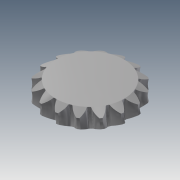
# Autodesk Inventor part: Worm Gear
Saved by Autodesk Inventor 2018 (Build 220112000, 112)
## iProperties
Created: 2019-02-07
Part Number: Worm Gear
Material: Steel, Mild
Document SubType Name: Modeling
Designer: Tsche
Categories: <?xml version="1.0" encoding="UTF-16"?> <MemberInstance><Categories><FamilyTemplate><FamilyTemplateParameter ValueType="xs:double" Id="1" ObjectReferenceKey="da_z" ObjectType="kUserParameterObject"/><FamilyTemplateParameter ValueType="xs:double" Id="2" ObjectReferenceKey="da_b" ObjectType="kUserParameterObject"/><FamilyTemplateParameter ValueType="xs:double" Id="3" ObjectReferenceKey="da_beta" ObjectType="kUserParameterObject"/><FamilyTemplateParameter ValueType="xs:double" Id="4" ObjectReferenceKey="da_m" ObjectType="kUserParameterObject"/><FamilyTemplateParameter ValueType="xs:double" Id="5" ObjectReferenceKey="da_alpha" ObjectType="kUserParameterObject"/><FamilyTemplateParameter ValueType="xs:double" Id="6" ObjectReferenceKey="da_da" ObjectType="kUserParameterObject"/><FamilyTemplateParameter ValueType="xs:double" Id="7" ObjectReferenceKey="da_aw" ObjectType="kUserParameterObject"/><FamilyTemplateParameter ValueType="xs:double" Id="8" ObjectReferenceKey="da_px" ObjectType="kUserParameterObject"/><FamilyTemplateParameter ValueType="xs:double" Id="9" ObjectReferenceKey="da_d" ObjectType="kUserParameterObject"/><FamilyTemplateParameter ValueType="xs:double" Id="10" ObjectReferenceKey="da_dae" ObjectType="kUserParameterObject"/><FamilyTemplateParameter ValueType="xs:double" Id="11" ObjectReferenceKey="da_fi" ObjectType="kUserParameterObject"/><FamilyTemplateParameter ValueType="xs:string" Id="12" ObjectReferenceKey="EAIAABAAAAAWFwAAAAAAAIAAAAAAAAAA" ObjectType="83910656" SubObjectId="SurfaceGeometry"/></FamilyTemplate><ParamToTemplateMap><ParamToTemplate CategoryParameter="//CategoryParameter[@InternalName='046C89C9-8512-4d59-83FE-43B91F4F132A']" TemplateParameter="1"/><ParamToTemplate CategoryParameter="//CategoryParameter[@InternalName='2552DF32-E462-4b46-AEBF-C6C7768E72AC']" TemplateParameter="2"/><ParamToTemplate CategoryParameter="//CategoryParameter[@InternalName='C9EE641D-15FC-4fae-A226-E94C4372FDD7']" TemplateParameter="3"/><ParamToTemplate><ParamToTemplate CategoryParameter="//CategoryParameter[@InternalName='00B6519A-459B-49c7-AD84-2E56D39A5744']" ConstantValue="0.000000"/></ParamToTemplate><ParamToTemplate><ParamToTemplate CategoryParameter="//CategoryParameter[@InternalName='04B31F0E-C7A6-4894-AA32-9629BEFACF47']" ConstantValue="1.000000"/></ParamToTemplate><ParamToTemplate><ParamToTemplate CategoryParameter="//CategoryParameter[@InternalName='43CBEC2E-7847-49e7-A936-2F7889FCB2D9']" ConstantValue="0.200000"/></ParamToTemplate><ParamToTemplate><ParamToTemplate CategoryParameter="//CategoryParameter[@InternalName='B1EFC894-105D-4ebd-86BF-FA20ED196853']" ConstantValue="0.300000"/></ParamToTemplate><ParamToTemplate><ParamToTemplate CategoryParameter="//CategoryParameter[@InternalName='51175063-3D10-4879-93E8-6246FE8B403D']" ConstantValue="2060000000.000000"/></ParamToTemplate><ParamToTemplate><ParamToTemplate CategoryParameter="//CategoryParameter[@InternalName='A3A52E27-4454-46a9-B0BD-C932399B70AF']" ConstantValue="0.300000"/></ParamToTemplate><ParamToTemplate CategoryParameter="//CategoryParameter[@InternalName='91B76062-C214-41d9-B1B9-14D2AB99603D']" TemplateParameter="4"/><ParamToTemplate CategoryParameter="//CategoryParameter[@InternalName='2D373A89-B862-43d6-8D0B-0CBF12AB9F6C']" TemplateParameter="5"/><ParamToTemplate CategoryParameter="//CategoryParameter[@InternalName='37777632-D6A2-4fac-9D53-DB8ACD95C989']" TemplateParameter="6"/><ParamToTemplate CategoryParameter="//CategoryParameter[@InternalName='FD1017F1-B727-4f7e-9707-0F86F1FF9423']" TemplateParameter="7"/><ParamToTemplate CategoryParameter="//CategoryParameter[@InternalName='3BF567DA-17EF-48d8-80EA-D119B07F6463']" TemplateParameter="8"/><ParamToTemplate CategoryParameter="//CategoryParameter[@InternalName='BF5A1E7E-5373-4a22-AAD3-F583781FCF3C']" TemplateParameter="9"/><ParamToTemplate CategoryParameter="//CategoryParameter[@InternalName='2A200944-5A8C-41ca-B96E-8520D2E510F1']" TemplateParameter="10"/><ParamToTemplate CategoryParameter="//CategoryParameter[@InternalName='E77AC4FD-7B43-4566-B0ED-7CA70B976BC8']" TemplateParameter="11"/><ParamToTemplate><ParamToTemplate CategoryParameter="//CategoryParameter[@InternalName='D4F72237-D604-435a-AD0B-F738B7463A00']" ConstantValue="110.000000"/></ParamToTemplate><ParamToTemplate><ParamToTemplate CategoryParameter="//CategoryParameter[@InternalName='9E1B4470-B2D3-4ff1-B813-535BB4CDF51A']" ConstantValue="2000000.000000"/></ParamToTemplate><ParamToTemplate><ParamToTemplate CategoryParameter="//CategoryParameter[@InternalName='A7A89E9A-52E6-4d4f-86CF-A81914F22AA4']" ConstantValue="250000000.000000"/></ParamToTemplate><ParamToTemplate><ParamToTemplate CategoryParameter="//CategoryParameter[@InternalName='B02FABAC-469F-4ad8-A219-DB4578299DF6']" ConstantValue="250000000.000000"/></ParamToTemplate><ParamToTemplate><ParamToTemplate CategoryParameter="//CategoryParameter[@InternalName='E6981962-40D5-4343-A0AD-C263FCC47E10']" ConstantValue="9.000000"/></ParamToTemplate><ParamToTemplate><ParamToTemplate CategoryParameter="//CategoryParameter[@InternalName='B958E99F-2BCD-4955-8634-793EB7B37B89']" ConstantValue="8.000000"/></ParamToTemplate><ParamToTemplate><ParamToTemplate CategoryParameter="//CategoryParameter[@InternalName='4AD49A87-569D-440f-A541-E3B52A6A9DCE']" ConstantValue="1200.000000"/></ParamToTemplate><ParamToTemplate><ParamToTemplate CategoryParameter="//CategoryParameter[@InternalName='4E5813A0-330D-4b41-BE23-D880B01A1D55']" ConstantValue="1650000.000000"/></ParamToTemplate><ParamToTemplate><ParamToTemplate CategoryParameter="//CategoryParameter[@InternalName='19EB8C86-AA88-4253-B4AA-2F5DF1CE171A']" ConstantValue="6000.000000"/></ParamToTemplate><ParamToTemplate CategoryParameter="//CategoryParameter[@InternalName='27C3BAF2-7550-4e4b-AE2C-0DB134B7D9B7']" TemplateParameter="12"/></ParamToTemplateMap><Category DisplayName="Gear" InternalName="DC85795E-93AB-48d5-8EEE-5A27447B64BD" Mnemonic="Gear"><CategoryParameter DisplayName="z" InternalName="046C89C9-8512-4d59-83FE-43B91F4F132A" Mnemonic="z"/><CategoryParameter DisplayName="b|.2|" InternalName="2552DF32-E462-4b46-AEBF-C6C7768E72AC" Mnemonic="b"/><CategoryParameter DisplayName="||b|" InternalName="C9EE641D-15FC-4fae-A226-E94C4372FDD7" Mnemonic="beta"/><CategoryParameter DisplayName="x" InternalName="00B6519A-459B-49c7-AD84-2E56D39A5744" Mnemonic="x"/><CategoryParameter DisplayName="a*" InternalName="04B31F0E-C7A6-4894-AA32-9629BEFACF47" Mnemonic="a"/><CategoryParameter DisplayName="c*" InternalName="43CBEC2E-7847-49e7-A936-2F7889FCB2D9" Mnemonic="c"/><CategoryParameter DisplayName="r|.f|*" InternalName="B1EFC894-105D-4ebd-86BF-FA20ED196853" Mnemonic="rf"/><CategoryParameter DisplayName="E" InternalName="51175063-3D10-4879-93E8-6246FE8B403D" Mnemonic="E"/><CategoryParameter DisplayName="||m|" InternalName="A3A52E27-4454-46a9-B0BD-C932399B70AF" Mnemonic="mi"/><Category DisplayName="WormGear" InternalName="1B25C7EF-093B-4025-B3D3-619CD2A4550C" Mnemonic="WormGear"><CategoryParameter DisplayName="m" InternalName="91B76062-C214-41d9-B1B9-14D2AB99603D" Mnemonic="m"/><CategoryParameter DisplayName="||a|" InternalName="2D373A89-B862-43d6-8D0B-0CBF12AB9F6C" Mnemonic="alpha"/><CategoryParameter DisplayName="d|.a|" InternalName="37777632-D6A2-4fac-9D53-DB8ACD95C989" Mnemonic="da"/><CategoryParameter DisplayName="a|.w|" InternalName="FD1017F1-B727-4f7e-9707-0F86F1FF9423" Mnemonic="aw"/><CategoryParameter DisplayName="p|.x|" InternalName="3BF567DA-17EF-48d8-80EA-D119B07F6463" Mnemonic="px"/><CategoryParameter DisplayName="d" InternalName="BF5A1E7E-5373-4a22-AAD3-F583781FCF3C" Mnemonic="d"/><CategoryParameter DisplayName="dae" InternalName="2A200944-5A8C-41ca-B96E-8520D2E510F1" Mnemonic="dae"/><CategoryParameter DisplayName="||d|" InternalName="E77AC4FD-7B43-4566-B0ED-7CA70B976BC8" Mnemonic="fi"/><CategoryParameter DisplayName="VHV" InternalName="D4F72237-D604-435a-AD0B-F738B7463A00" Mnemonic="VHV"/><CategoryParameter DisplayName="||s||.Hlim|" InternalName="9E1B4470-B2D3-4ff1-B813-535BB4CDF51A" Mnemonic="sHlim"/><CategoryParameter DisplayName="N|.Flim|" InternalName="A7A89E9A-52E6-4d4f-86CF-A81914F22AA4" Mnemonic="NFlim"/><CategoryParameter DisplayName="N|.Hlim|" InternalName="B02FABAC-469F-4ad8-A219-DB4578299DF6" Mnemonic="NHlim"/><CategoryParameter DisplayName="q|.F|" InternalName="E6981962-40D5-4343-A0AD-C263FCC47E10" Mnemonic="qF"/><CategoryParameter DisplayName="q|.H|" InternalName="B958E99F-2BCD-4955-8634-793EB7B37B89" Mnemonic="qH"/><CategoryParameter DisplayName="v|.max|" InternalName="4AD49A87-569D-440f-A541-E3B52A6A9DCE" Mnemonic="maxv"/><CategoryParameter DisplayName="S|.n|" InternalName="4E5813A0-330D-4b41-BE23-D880B01A1D55" Mnemonic="Sn"/><CategoryParameter DisplayName="K|.w|" InternalName="19EB8C86-AA88-4253-B4AA-2F5DF1CE171A" Mnemonic="Kw"/><CategoryParameter DisplayName="PitchDiameter" InternalName="27C3BAF2-7550-4e4b-AE2C-0DB134B7D9B7" Mnemonic="IDS_PITCHDIAM"/></Category></Category></Categories></MemberInstance>
Density: 7.86 g/cm^3
Appearance: Steel
CustomPartVersion: 1
Author: Tsche
Autodesk Inventor part; units mm, degrees
sketch "Sketch9" plane through (0, 0, 0) normal (0, 0, 1) x (1, 0, 0)
  spline S0 degree 4 poles (-1.8496, 10.8434) (-1.7998, 10.7978) (-1.7009, 10.7058) (-1.5459, 10.5544) (-1.3329, 10.3239) (-1.1209, 10.0648) (-0.9158, 9.786) (-0.7302, 9.464) (-0.6035, 9.2436) (-0.4689, 8.8382) (-0.423, 8.7684) (-0.3393, 8.6727) (-0.2622, 8.6399) (-0.1993, 8.6478) (-0.1698, 8.6483) knots 0 0 0 0 0 0.083363 0.166726 0.277875 0.389023 0.500167 0.611302 0.70854 0.791872 0.861267 0.916769 1 1 1 1 1
  line L0 (-0.5286, 8.6413) -> (0.1889, 8.6554) construction
  arc A0 (0.0361, 8.5685) -> (-0.3725, 8.5605) centre (-0.1641, 8.3574) ccw construction
  circle A1 centre (0, 0) radius 8.65 construction
  circle A2 centre (0, 0) radius 8.6603 construction
  circle A3 centre (0, 0) radius 10 construction
  circle A4 centre (0, 0) radius 11 construction
  line L1 (0, 0) -> (0, 11) construction
  line L2 (-0.216, 10.9979) -> (0, 0) construction
  line L3 (-1.8496, 10.8434) -> (-2.5, 11.4389)
  line L4 (-2.1516, 11.1199) -> (-1.5476, 10.5669) construction
  arc A5 (-1.6113, 10.6188) -> (-2.0943, 11.061) centre (-9.4861, 2.5022) ccw construction
  line L5 (-2.5, 11.4389) -> (-2.5, 12.998)
  line L6 (-2.5, 12.998) -> (0, 12.998)
  arc A6 (0, 8.65) -> (-0.1698, 8.6483) centre (0, 0) ccw
  line L7 (1.8496, 10.8434) -> (2.5, 11.4389)
  line L8 (2.5, 11.4389) -> (2.5, 12.998)
  line L9 (2.5, 12.998) -> (0, 12.998)
  arc A7 (0.1698, 8.6483) -> (0, 8.65) centre (0, 0) ccw
  spline S1 degree 4 poles (1.8496, 10.8434) (1.7998, 10.7978) (1.7009, 10.7058) (1.5459, 10.5544) (1.3329, 10.3239) (1.1209, 10.0648) (0.9158, 9.786) (0.7302, 9.464) (0.6035, 9.2436) (0.4689, 8.8382) (0.423, 8.7684) (0.3393, 8.6727) (0.2622, 8.6399) (0.1993, 8.6478) (0.1698, 8.6483) knots 0 0 0 0 0 0.083363 0.166726 0.277875 0.389023 0.500167 0.611302 0.70854 0.791872 0.861267 0.916769 1 1 1 1 1
  line L10 (0.5286, 8.6413) -> (-0.1889, 8.6554) construction
  line L11 (2.1516, 11.1199) -> (1.5476, 10.5669) construction
  arc A8 (0.3725, 8.5605) -> (-0.0361, 8.5685) centre (0.1641, 8.3574) ccw construction
  arc A9 (2.0943, 11.061) -> (1.6113, 10.6188) centre (9.4861, 2.5022) ccw construction
  line L12 (-2.5, 12.998) -> (-2.5, 17) construction
  line L13 (-2.5, 17) -> (2.5, 17) construction
  line L14 (2.5, 17) -> (2.5, 12.998) construction
  constraints: 1 other
ref_plane "Tooth Plane" through (0, -10, 0) normal (-0.071247, 0, 0.9974587) x (0, 1, 0)
sketch "Base Body Sketch" plane through (0, 0, 0) normal (1, 0, 0) x (0, 1, 0)
  line L0 (0, -8.4) -> (0, 8.4) projected
  line L1 (0, 2.5) -> (9.035, 2.5)
  line L2 (9.035, 2.5) -> (11.5, 1.0768)
  line L3 (-4.6, 0) -> (27.6, 0) construction
  circle A0 centre (17, 0) radius 6
  line L4 (11.5, 1.0768) -> (11.5, -1.0768)
  line L5 (0, -2.5) -> (9.035, -2.5)
  line L6 (0, 2.5) -> (0, -2.5)
  line L7 (9.035, -2.5) -> (11.5, -1.0768)
  dimension "d87" = 23
  dimension "d89" = 12
  dimension "d92" = 5
  dimension "d93" = 17
  dimension "d119" = 30
  dimension "d122" = 9.035
  constraints: 14 end point, 3 symmetric about line, 2 perpendicular, 1 centre point, 1 collinear, 1 point on line
  measures "d87" diameter of L4 L0
  measures "d89" diameter of A0
  measures "d92" distance of L1.start L5.start
  measures "d93" distance from line of A0.centre L6
  measures "d119" angle of L1 L2
  measures "d122" distance of L1.start L1.end
revolve "Base Body" add sketch "Base Body Sketch" angle 360 about axis through (0, 0, 0) along (0, 0, 1) picked at (11.3385, 0.1438) contours L0 L1 L2 A0 L7 L5 | A0 L2 L4 L7
revolve "Base Body2" cut sketch "Base Body Sketch" angle 360 about axis through (0, 0, 0) along (0, 0, 1) contours L7 L4 L2 A0 | A0 L2 L4 L7
sketch "Tooth Sketch" plane through (0, -10, 0) normal (-0.071247, 0, 0.9974587) x (0, 1, 0)
  line L0 (10, 2.2608) -> (10, -2.2608) projected
  line L1 (-8.64, 0) -> (2.84, 0) projected
  line L2 (-7, 1.6149) -> (-7, -1.6149)
  line L3 (-7, -1.6149) -> (-1.2, -1.6149)
  line L4 (-1.2, -1.6149) -> (1.2, -0.7413)
  line L5 (1.2, -0.7413) -> (1.2, 0)
  line L6 (1.2, 0.7413) -> (-1.2, 1.6149)
  line L7 (-1.2, 1.6149) -> (-7, 1.6149)
  line L8 (1.2, 0.7413) -> (1.2, 0)
  line L9 (0, 0) -> (0, -1.1781) construction
  dimension "d38" = 17
  dimension "d39" = 20
  dimension "d40" = 5.8
  dimension "d41" = 7
  dimension "d42" = 1.1781
  constraints: 16 end point, 4 perpendicular, 3 equal length, 2 point on line, 1 midpoint, 1 parallel, 1 vertical
  measures "d38" distance between parallel lines of L0 L2
  measures "d39" angle of L6 L7
  measures "d40" distance of L6.end L2.start
  measures "d41" distance between parallel lines of L2 L9
  measures "d42" distance of L9.start L9.end
sketch "Sketch8" plane through (0, 0, 2.5) normal (0, 0, 1) x (1, 0, 0)
  circle A0 centre (0, 0) radius 9.035 projected
  circle A1 centre (0, 0) radius 10
  dimension "d77" = 20
  constraints: 1 centre point, 1 coincident
  measures "d77" diameter of A1
sketch "involute_tooth" plane through (0, 0, 0) normal (0, 0, 1) x (1, 0, 0)
  spline S0 degree 4 poles (-1.6363, 10.8776) (-1.5874, 10.831) (-1.4904, 10.7371) (-1.3384, 10.5827) (-1.1299, 10.3481) (-0.9231, 10.0849) (-0.7235, 9.8021) (-0.5442, 9.4765) (-0.4219, 9.2536) (-0.2952, 8.8457) (-0.2508, 8.775) (-0.169, 8.6777) (-0.0925, 8.6433) (-0.0295, 8.65) (0, 8.65) knots 0 0 0 0 0 0.083363 0.166726 0.277875 0.389023 0.500167 0.611302 0.70854 0.791872 0.861267 0.916769 1 1 1 1 1
  line L0 (-0.3588, 8.65) -> (0.3588, 8.65) construction
  arc A0 (0.2043, 8.5662) -> (-0.2043, 8.5662) centre (0, 8.359) ccw construction
  circle A1 centre (0, 0) radius 8.65 construction
  circle A2 centre (0, 0) radius 8.6603 construction
  circle A3 centre (0, 0) radius 10 construction
  circle A4 centre (0, 0) radius 11 construction
  line L1 (0, 0) -> (0.216, 10.9979) construction
  line L2 (0, 11) -> (0, 0) construction
  line L3 (-1.6363, 10.8776) -> (-2.2749, 11.4857)
  line L4 (-1.9329, 11.16) -> (-1.3398, 10.5952) construction
  arc A5 (-1.4025, 10.6484) -> (-1.8767, 11.1) centre (-9.4352, 2.688) ccw construction
  line L5 (-2.2749, 11.4857) -> (-2.2443, 13.0446)
  line L6 (-2.2443, 13.0446) -> (0.2552, 12.9955)
  arc A6 (0.1698, 8.6483) -> (0, 8.65) centre (0, 0) ccw
  line L7 (2.0621, 10.805) -> (2.7241, 11.3876)
  line L8 (2.7241, 11.3876) -> (2.7547, 12.9464)
  line L9 (2.7547, 12.9464) -> (0.2552, 12.9955)
  arc A7 (0.3396, 8.6433) -> (0.1698, 8.6483) centre (0, 0) ccw
  spline S1 degree 4 poles (2.0621, 10.805) (2.0114, 10.7604) (1.9108, 10.6704) (1.7529, 10.522) (1.5353, 10.2958) (1.3183, 10.0408) (1.1078, 9.7662) (0.9158, 9.4479) (0.7848, 9.2299) (0.6423, 8.8273) (0.5951, 8.7584) (0.5095, 8.6644) (0.4318, 8.633) (0.3691, 8.6422) (0.3396, 8.6433) knots 0 0 0 0 0 0.083363 0.166726 0.277875 0.389023 0.500167 0.611302 0.70854 0.791872 0.861267 0.916769 1 1 1 1 1
  line L10 (0.6981, 8.6292) -> (-0.0189, 8.6574) construction
  line L11 (2.3695, 11.0755) -> (1.7547, 10.5345) construction
  arc A8 (0.5405, 8.5515) -> (0.1321, 8.5676) centre (0.3282, 8.3526) ccw construction
  arc A9 (2.3111, 11.0178) -> (1.8194, 10.5851) centre (9.5334, 2.3155) ccw construction
  line L12 (-2.2443, 13.0446) -> (-2.1657, 17.0458) construction
  line L13 (-2.1657, 17.0458) -> (2.8333, 16.9476) construction
  line L14 (2.8333, 16.9476) -> (2.7547, 12.9464) construction
  point P0 (0.3349, 9.3778)
  point P1 (-1.1477, 10.3628)
  point P2 (-0.9274, 10.0843)
  point P3 (-0.7266, 9.7915)
  point P4 (-0.549, 9.4841)
  point P5 (-0.4003, 9.1618)
  point P6 (-0.2776, 8.8289)
  point P7 (-0.2307, 8.7536)
  point P8 (-0.1685, 8.6905)
  point P9 (-0.0886, 8.6532)
  point P10 (1.5536, 10.3097)
  point P11 (1.3226, 10.0401)
  point P12 (1.1105, 9.7554)
  point P13 (0.9209, 9.4553)
  point P14 (0.7597, 9.139)
  point P15 (0.624, 8.8112)
  point P16 (0.5742, 8.7378)
  point P17 (0.5096, 8.6772)
  point P18 (0.4283, 8.6431)
  dimension "d97" = 1.125
  dimension "d98" = 2.5
  dimension "d99" = 17
  constraints: 30 end point, 24 symmetric about line, 15 point on circle, 9 centre point, 6 midpoint, 3 collinear, 2 horizontal, 2 parallel, 2 point on line, 1 coincident, 1 perpendicular, 1 tangent, 1 vertical, 54 other
  measures "d97" angle of L2 L1
  measures "d98" distance between parallel lines of L1 L5
  measures "d99" distance from line of point (0, 0) L13
surface extrude "Pitch Diameter" sketch "Sketch8" against normal blind 5 shown no curves A1
ref_plane "Work Plane13" through (0, 0, 0) normal (-0.1564345, 0.9876883, 0) x (0, 0, 1)
revolve "Tooth" [suppressed]
pattern_circular "Tooth Pattern" [suppressed]
ref_plane "Work Plane14" through (0, 0, 0) normal (0.9876883, 0.1564345, 0) x (0, 0, 1)
ref_plane "Work Plane15" through (0, 0, 0) normal (0, -1, 0) x (0, 0, 1)
coil "Coil1" sketch "Sketch9" operation cut axis through (-2.5, 17, 0) along (-1, 0, 0) pitch 3.927 turns 0.5 hand left
coil "Coil2" sketch "Sketch9" operation cut axis through (-2.5, 17, 0) along (1, 0, 0) pitch 3.927 turns 0.5 hand left
pattern_circular "Circular Pattern2" count 16 over 360 about axis through (0, 0, 0) along (0, 0, 1) of "Coil1", "Coil2"
equation "\"d87\" = da_dae"
equation "\"d89\" = 2 * da_aw - da_da"
equation "\"d92\" = da_b"
equation "\"d93\" = da_aw"
equation "\"d119\" = da_fi"
equation "\"d99\" = da_aw"
equation "\"d100\" = da_px"
equation "\"d111\" = da_px"
equation "\"d38\" = da_aw"
equation "\"d39\" = da_alfat"
equation "\"d40\" = 0.5 * da_df1"
equation "\"d41\" = 0.5 * da_d1"
equation "\"d42\" = 0.3 * da_px"
equation "\"d77\" = da_dw"
equation "\"d78\" = da_b"
equation "\"da_aw\" = 17"
equation "\"da_fi\" = 30deg"
equation "\"da_b\" = 5"
equation "\"da_df\" = 17.6"
equation "\"da_da\" = 22"
equation "\"da_beta\" = 4.085617deg"
equation "\"da_alfat\" = 20deg"
equation "\"da_df1\" = 11.6"
equation "\"da_da1\" = 16"
equation "\"da_d1\" = 14"
equation "\"da_px\" = 3.92699"
equation "\"d68\" = da_aw"
equation "\"da_dw\" = 20"
equation "\"da_rightdir\" = 0"
equation "\"d86\" = da_aw"
equation "\"da_dae\" = 23"
body "Solid1"
body "Srf1"
